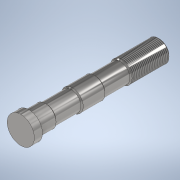
# Autodesk Inventor part: Болт шатуна
Saved by Autodesk Inventor 2021 (Build 250183000, 183)
## iProperties
Created: 2020-12-21
Part Number: Болт шатуна
Material: Сталь, высокопрочная, низколегированная
Document SubType Name: Modeling
Designer: Тимоха
Mass: 2416.74 g
Surface Area: 354.793 cm^2
Volume: 307.865 cm^3
Density: 7.85 g/cm^3
Appearance: Сталь — полированная
Author: Тимоха
Autodesk Inventor part; units mm, degrees
ref_plane "YZ Plane" through (0, 0, 0) normal (1, 0, 0) x (0, 1, 0)
ref_plane "XZ Plane" through (0, 0, 0) normal (0, 1, 0) x (-1, 0, 0)
ref_plane "XY Plane" through (0, 0, 0) normal (0, 0, 1) x (1, 0, 0)
sketch "Эскиз1" plane through (0, 0, 0) normal (0, 0, 1) x (1, 0, 0)
  circle A0 centre (0, 0) radius 25
  dimension "d0" = 50
  constraints: 1 centre point, 1 coincident
  measures "d0" diameter of A0
extrude "Выдавливание1" add sketch "Эскиз1" along normal blind 15
sketch "Эскиз2" plane through (0, 0, 0) normal (0, 0, -1) x (-1, 0, 0)
  circle A0 centre (0, 0) radius 25 projected
  circle A1 centre (0, 0) radius 20
  dimension "d3" = 40
  constraints: 1 centre point, 1 coincident
  measures "d3" diameter of A1
extrude "Выдавливание2" add sketch "Эскиз2" along normal blind 200 contours A1
sketch "Эскиз3" plane through (0, 0, 0) normal (1, 0, 0) x (0, 1, 0)
  line L0 (-20, -200) -> (20, -200) projected
  line L1 (20, 0) -> (-20, 0) projected
  line L2 (20, 0) -> (20, -200) projected
  line L3 (-20, 0) -> (-20, -200) projected
  line L4 (20, 0) -> (20, -30)
  line L5 (20, -30) -> (20, -30)
  line L6 (18, -32) -> (18, -78)
  line L7 (20, -80) -> (20, -80)
  line L8 (20, -80) -> (20, -120)
  line L9 (20, -120) -> (20, -120)
  line L10 (18, -122) -> (18, -168)
  line L11 (20, -170) -> (20, -170)
  line L12 (20, -30) -> (18, -32)
  line L13 (18, -78) -> (20, -80)
  line L14 (20, -120) -> (18, -122)
  line L15 (18, -168) -> (20, -170)
  line L16 (0, 0) -> (0, -14)
  point P0 (18, -30)
  point P1 (18, -80)
  point P2 (18, -120)
  point P3 (18, -170)
  dimension "d6" = 30
  dimension "d7" = 2
  dimension "d8" = 50
  dimension "d9" = 40
  dimension "d10" = 50
  dimension "d11" = 2
  dimension "d12" = 2
  dimension "d13" = 2
  dimension "d14" = 2
  dimension "d15" = 2
  dimension "d16" = 2
  dimension "d17" = 2
  dimension "d18" = 2
  constraints: 26 end point, 12 point on line, 5 perpendicular, 1 parallel, 1 vertical
  measures "d6" distance of L2.start L4.end
  measures "d7" distance of L4.end point (18, -30)
  measures "d8" distance of point (18, -30) point (18, -80)
  measures "d9" distance of L7.end L8.end
  measures "d10" distance of point (18, -120) point (18, -170)
  measures "d11" distance of L5.end point (18, -30)
  measures "d12" distance of L6.start point (18, -30)
  measures "d13" distance of L6.end point (18, -80)
  measures "d14" distance of L7.start point (18, -80)
  measures "d15" distance of L9.end point (18, -120)
  measures "d16" distance of L10.start point (18, -120)
  measures "d17" distance of L10.end point (18, -170)
  measures "d18" distance of L11.start point (18, -170)
revolve "Вращение1" cut sketch "Эскиз3" angle 360 about axis through (0, 0, 0) along (0, 0, -1) contours L15 L10 L14 L2 | L13 L6 L12 L2
sketch "Эскиз4" plane through (0, 0, -200) normal (0, 0, -1) x (-1, 0, 0)
  circle A0 centre (0, 0) radius 20 projected
extrude "Выдавливание3" add sketch "Эскиз4" along normal blind 40
thread "Резьба1" size "M40x3" class "6g" standard "ANSI Metric M Profile" full length
chamfer "Фаска1" distance 2 angle 45 1 edges at (20, 0, -240)
equation "\"d12\" = d11"
equation "\"d13\" = d11"
equation "\"d14\" = d13"
equation "\"d15\" = d11"
equation "\"d16\" = d15"
equation "\"d17\" = d11"
equation "\"d18\" = d17"
